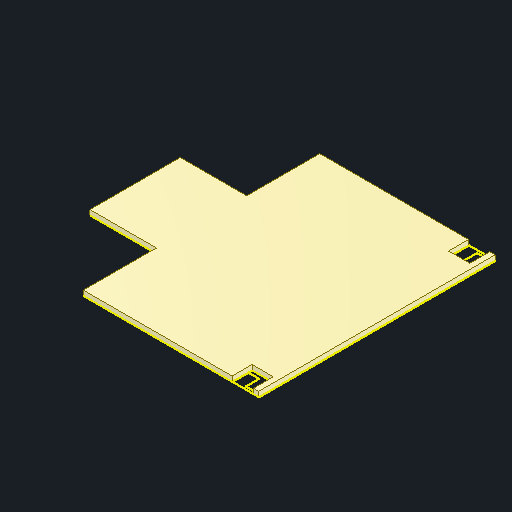
# Autodesk Inventor part: base
Saved by Autodesk Inventor 2023 (Build 270158000, 158)
## iProperties
Created: 2024-04-29
Part Number: base
Material: Nylon 6/6
Document SubType Name: Modeling
Designer: szymo
Density: 1.13 g/cm^3
Appearance: Nylon 6
Mass: 104.475 g
Surface Area: 555.62 cm^2
Volume: 92.456 cm^3
Author: szymo
Autodesk Inventor part; units mm, degrees
ref_plane "YZ Plane" through (0, 0, 0) normal (1, 0, 0) x (0, 1, 0)
ref_plane "XZ Plane" through (0, 0, 0) normal (0, 1, 0) x (-1, 0, 0)
ref_plane "XY Plane" through (0, 0, 0) normal (0, 0, 1) x (1, 0, 0)
sketch "Sketch1" plane through (0, 0, 0) normal (0, 1, 0) x (-1, 0, 0)
  line L0 (99, 89) -> (-99, 89)
  line L1 (-99, 89) -> (-99, -89)
  line L2 (-99, -89) -> (99, -89)
  line L3 (99, -89) -> (99, 89)
  line L4 (99, 89) -> (-99, -89) construction
  line L5 (-99, 89) -> (99, -89) construction
  line L6 (-99, 89) -> (-85, 89)
  line L7 (-85, 89) -> (-85, -89)
  line L8 (-85, -89) -> (-99, -89)
  line L9 (-99, -89) -> (-99, 89)
  line L10 (99, 89) -> (97, 89)
  line L11 (97, 89) -> (97, -89)
  line L12 (97, -89) -> (99, -89)
  line L13 (99, -89) -> (99, 89)
  line L14 (97, 33) -> (97, 35)
  line L15 (97, -33) -> (97, -35)
  line L16 (97, 32.8) -> (97, 35)
  line L17 (97, -32.8) -> (97, -35)
  line L18 (97, 89) -> (47, 89)
  line L19 (47, 89) -> (47, 34)
  line L20 (47, 34) -> (97, 34)
  line L21 (97, 34) -> (97, 89)
  line L22 (97, -89) -> (47, -89)
  line L23 (47, -89) -> (47, -34)
  line L24 (47, -34) -> (97, -34)
  line L25 (97, -34) -> (97, -89)
  line L26 (66.5, 33) -> (77.5, 33) projected
  line L27 (77.5, -33) -> (66.5, -33) projected
  line L28 (-81, 74) -> (-81, 89) projected
  line L29 (-81, 31) -> (-81, 55) projected
  line L30 (-81, -12) -> (-81, 12) projected
  line L31 (-81, -55) -> (-81, -31) projected
  line L32 (-81, -89) -> (-81, -74) projected
  arc A0 (-81, 74) -> (-79, 72) centre (-79, 74) ccw projected
  line L33 (-70, 72) -> (-79, 72) projected
  line L34 (-70, 57) -> (-70, 72) projected
  line L35 (-79, 57) -> (-70, 57) projected
  arc A1 (-79, 57) -> (-81, 55) centre (-79, 55) ccw projected
  arc A2 (-81, 31) -> (-79, 29) centre (-79, 31) ccw projected
  line L36 (-70, 29) -> (-79, 29) projected
  line L37 (-70, 14) -> (-70, 29) projected
  line L38 (-79, 14) -> (-70, 14) projected
  arc A3 (-79, 14) -> (-81, 12) centre (-79, 12) ccw projected
  arc A4 (-81, -12) -> (-79, -14) centre (-79, -12) ccw projected
  line L39 (-70, -14) -> (-79, -14) projected
  line L40 (-70, -29) -> (-70, -14) projected
  line L41 (-79, -29) -> (-70, -29) projected
  arc A5 (-79, -29) -> (-81, -31) centre (-79, -31) ccw projected
  arc A6 (-81, -55) -> (-79, -57) centre (-79, -55) ccw projected
  line L42 (-70, -57) -> (-79, -57) projected
  line L43 (-70, -72) -> (-70, -57) projected
  line L44 (-79, -72) -> (-70, -72) projected
  arc A7 (-79, -72) -> (-81, -74) centre (-79, -74) ccw projected
  circle A8 centre (-77, -64.5) radius 1.2295 projected
  circle A9 centre (-77, -21.5) radius 1.2295 projected
  circle A10 centre (-77, 21.5) radius 1.2295 projected
  circle A11 centre (-77, 64.5) radius 1.2295 projected
  line L45 (-65, 89) -> (-79, 89)
  line L46 (-79, 89) -> (-79, 75)
  line L47 (-79, 75) -> (-65, 75)
  line L48 (-65, 75) -> (-65, 89)
  line L49 (-65, 89) -> (-81, 89)
  line L50 (-81, 89) -> (-81, 74)
  line L51 (-81, 74) -> (-65, 74)
  line L52 (-65, 74) -> (-65, 89)
  line L53 (-99, 0) -> (97, 0)
  line L54 (0, 0) -> (-99, 0) construction
  line L55 (-65, -89) -> (-79, -89)
  line L56 (-79, -89) -> (-79, -75)
  line L57 (-79, -75) -> (-65, -75)
  line L58 (-65, -75) -> (-65, -89)
  line L59 (-65, -89) -> (-81, -89)
  line L60 (-81, -89) -> (-81, -74)
  line L61 (-81, -74) -> (-65, -74)
  line L62 (-65, -74) -> (-65, -89)
  point P0 (47, 89)
  point P1 (47, -89)
  point P2 (97, 34)
  point P3 (-81, -89)
  point P4 (-79, -74)
  dimension "d0" = 198
  dimension "d1" = 178
  dimension "d2" = 14
  dimension "d3" = 2
  dimension "d16" = 50
  dimension "d17" = 55
  dimension "d18" = 50
  dimension "d19" = 55
  dimension "d20" = 1
  dimension "d21" = 1
  dimension "d22" = 14
  dimension "d23" = 14
  dimension "d24" = 2
  dimension "d25" = 1
  dimension "d26" = 2
  constraints: 88 end point, 14 parallel, 10 symmetric about line, 8 perpendicular, 8 point on line, 7 horizontal, 4 midpoint, 2 collinear
  measures "d0" distance of L2.end L1.end
  measures "d1" distance of L1.end L0.end
  measures "d2" distance of L7.end L8.end
  measures "d3" distance of L12.end L11.end
  measures "d16" distance of L20.end L19.end
  measures "d17" distance of L19.end L18.end
  measures "d18" distance of L23.end L24.end
  measures "d19" distance of L22.end L23.end
  measures "d20" distance between parallel lines of L20 L26
  measures "d21" distance between parallel lines of L27 L24
  measures "d22" distance of L47.end L46.end
  measures "d23" distance of L46.end L45.end
  measures "d24" distance between parallel lines of L28 L46
  measures "d25" distance between parallel lines of L47 L51
  measures "d26" distance between parallel lines of L33 L51
extrude "Extrusion1" add sketch "Sketch1" along normal blind 3.5 contours L19 L20 L11 L53 L30 A3 L38 L37 L36 A2 L29 A1 L35 L34 L33 A0 L51 L52 L48 L0 | L2 L58 L62 L61 A7 L44 L43 L42 A6 L31 A5 L41 L40 L39 A4 L30 L53 L11 L24 L23 | L28 A0 L33 L34 L35 A1 L29 A2 L36 L37 L38 A3 L30 L53 L7 L0 | L2 L7 L53 L30 A4 L39 L40 L41 A5 L31 A6 L42 L43 L44 A7 L32 | A8 | A9 | A10 | A11
sketch "Sketch2" plane through (0, 0, 0) normal (0, -1, 0) x (1, 0, 0)
  line L0 (65, -74) -> (65, -89) projected
  line L1 (81, -74) -> (65, -74) projected
  line L2 (81, -89) -> (81, -74) projected
  line L3 (85, -89) -> (81, -89) projected
  line L4 (85, 89) -> (85, -89) projected
  line L5 (81, 89) -> (85, 89) projected
  line L6 (81, 74) -> (81, 89) projected
  line L7 (65, 74) -> (81, 74) projected
  line L8 (65, 89) -> (65, 74) projected
  line L9 (-47, 89) -> (65, 89) projected
  line L10 (-47, 34) -> (-47, 89) projected
  line L11 (-97, 34) -> (-47, 34) projected
  line L12 (-97, -34) -> (-97, 34) projected
  line L13 (-47, -34) -> (-97, -34) projected
  line L14 (-47, -89) -> (-47, -34) projected
  line L15 (65, -89) -> (-47, -89) projected
  circle A0 centre (61.5, -80) radius 1.8 projected
  circle A1 centre (-18.3706, -84.6) radius 1.8 projected
  line L16 (81, -87) -> (73, -87) projected
  line L17 (73, -87) -> (73, -77) projected
  line L18 (73, -77) -> (58, -77) projected
  line L19 (58, -77) -> (58, -83) projected
  line L20 (58, -83) -> (-14.925, -83) projected
  line L21 (-14.925, -83) -> (-14.925, -70.4) projected
  line L22 (-14.925, -70.4) -> (-47, -70.4) projected
  line L23 (-47, -89) -> (-47, -70.4) projected
  line L24 (-47, -89) -> (81, -89) projected
  line L25 (81, -89) -> (81, -87) projected
  circle A2 centre (61.5, 80) radius 1.8 projected
  circle A3 centre (-18.3706, 84.6) radius 1.8 projected
  line L26 (81, 87) -> (73, 87) projected
  line L27 (81, 89) -> (81, 87) projected
  line L28 (-47, 89) -> (81, 89) projected
  line L29 (-47, 89) -> (-47, 70.4) projected
  line L30 (-14.925, 70.4) -> (-47, 70.4) projected
  line L31 (-14.925, 83) -> (-14.925, 70.4) projected
  line L32 (58, 83) -> (-14.925, 83) projected
  line L33 (58, 77) -> (58, 83) projected
  line L34 (73, 77) -> (58, 77) projected
  line L35 (73, 87) -> (73, 77) projected
  line L36 (69.5, -34) -> (69.5, -27) projected
  line L37 (69.5, -27) -> (-97, -27) projected
  line L38 (-97, -27) -> (-97, -34) projected
  line L39 (-97, -34) -> (-94, -34) projected
  line L40 (-94, -34) -> (41.0514, -34) projected
  line L41 (41.0514, -34) -> (41.0514, -45) projected
  line L42 (41.0514, -45) -> (45.7494, -45) projected
  line L43 (45.7494, -45) -> (45.7494, -34.8203) projected
  line L44 (45.7494, -45) -> (59.075, -45) projected
  line L45 (59.075, -34) -> (59.075, -45) projected
  line L46 (59.075, -34) -> (69.5, -34) projected
  line L47 (69.5, 34) -> (69.5, 27) projected
  line L48 (59.075, 34) -> (69.5, 34) projected
  line L49 (59.075, 34) -> (59.075, 45) projected
  line L50 (45.7494, 45) -> (59.075, 45) projected
  line L51 (45.7494, 45) -> (45.7494, 34.8203) projected
  line L52 (41.0514, 45) -> (45.7494, 45) projected
  line L53 (41.0514, 34) -> (41.0514, 45) projected
  line L54 (-94, 34) -> (41.0514, 34) projected
  line L55 (-97, 34) -> (-94, 34) projected
  line L56 (-97, 27) -> (-97, 34) projected
  line L57 (69.5, 27) -> (-97, 27) projected
  circle A4 centre (-56.325, 30.5) radius 1.8 projected
  circle A5 centre (-56.325, -30.5) radius 1.8 projected
  circle A6 centre (66.25, 30.5) radius 1.8 projected
  circle A7 centre (66.25, -30.5) radius 1.8 projected
  point P0 (0, 0)
body "Solid1"
